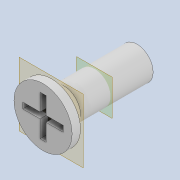
# Autodesk Inventor part: m2 screw
Saved by Autodesk Inventor 2022.3 (Build 263350030, 350C)
## iProperties
Created: 2022-11-02
Part Number: m2 screw
Material: Generic
Document SubType Name: Modeling
Designer: benka
Density: 1 g/cm^3
Appearance: Default
Author: benka
Autodesk Inventor part; units mm, degrees
ref_plane "YZ Plane" through (0, 0, 0) normal (1, 0, 0) x (0, 1, 0)
ref_plane "XZ Plane" through (0, 0, 0) normal (0, 1, 0) x (-1, 0, 0)
ref_plane "XY Plane" through (0, 0, 0) normal (0, 0, 1) x (1, 0, 0)
sketch "Sketch1" plane through (0, 0, 0) normal (0, 0, 1) x (1, 0, 0)
  ellipse E0 centre (-142.8213, 11.369) end of major axis (-142.8213, 12.3754) minor radius 1
  point P0 (0, 0)
  dimension "d1" = 1.0064
  constraints: 2 other
extrude "Extrusion1" add sketch "Sketch1" against normal blind 4.5
sketch "Sketch2" plane through (0, 0, 0) normal (0, 0, 1) x (1, 0, 0)
  ellipse E0 centre (-142.8213, 11.369) end of major axis (-142.8213, 12.3754) minor radius 1 projected
  circle A0 centre (-142.8213, 11.369) radius 1.8
  point P0 (0, 0)
  dimension "d4" = 3.6
  constraints: 1 centre point, 1 coincident, 1 other
  measures "d4" diameter of A0
extrude "Extrusion2" add sketch "Sketch2" along normal blind 1.32 contours E0 | A0
ref_plane "Work Plane1" through (-142.8213, 11.369, 0.82) normal (0, 0, 1) x (1, 0, 0)
chamfer "Chamfer1" distance 0.7999 angle 45 1 edges at (-144.6213, 11.369, 0)
sketch "Sketch3" plane through (-142.8213, 11.369, 1.32) normal (0, 0, 1) x (1, 0, 0)
  line L0 (0, 0) -> (0, -1.25)
  line L1 (0, 0) -> (0, 1.25)
  line L2 (0, 0) -> (1.25, 0)
  line L3 (1.25, 0) -> (-1.25, 0)
  line L4 (-1.25, -0.1847) -> (1.25, -0.1847)
  line L5 (1.25, -0.1847) -> (1.25, 0.1847)
  line L6 (1.25, 0.1847) -> (-1.25, 0.1847)
  line L7 (-1.25, 0.1847) -> (-1.25, -0.1847)
  line L8 (-1.25, -0.1847) -> (1.25, 0.1847) construction
  line L9 (1.25, -0.1847) -> (-1.25, 0.1847) construction
  line L10 (-0.1847, -1.25) -> (0.1847, -1.25)
  line L11 (0.1847, -1.25) -> (0.1847, 1.25)
  line L12 (0.1847, 1.25) -> (-0.1847, 1.25)
  line L13 (-0.1847, 1.25) -> (-0.1847, -1.25)
  line L14 (-0.1847, -1.25) -> (0.1847, 1.25) construction
  line L15 (0.1847, -1.25) -> (-0.1847, 1.25) construction
  point P0 (142.8213, -11.369)
  point P1 (0.1847, 0.1847)
  point P2 (-0.1847, 0.1847)
  point P3 (-0.1847, -0.1847)
  point P4 (0.1847, -0.1847)
  dimension "d11" = 1.25
  dimension "d12" = 1.25
  dimension "d13" = 1.25
  dimension "d14" = 2.5
  constraints: 32 end point, 4 midpoint, 4 parallel, 2 horizontal, 2 perpendicular, 1 point on line, 1 vertical
  measures "d11" distance of L0.start L0.end
  measures "d12" distance of L0.start L1.end
  measures "d13" distance of L2.start L2.end
  measures "d14" distance of L2.end L3.end
extrude "Extrusion3" cut sketch "Sketch3" against normal blind 0.5
ref_plane "Work Plane2" through (0, 0, -1.86) normal (0, 0, -1) x (-1, 0, 0)
body "Solid1"
